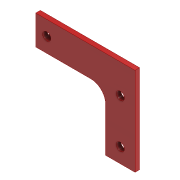
# Autodesk Inventor part: Odometry stop
Saved by Autodesk Inventor 2020 (Build 240168000, 168)
## iProperties
Created: 2020-03-07
Part Number: Odometry stop
Material: Generic
Document SubType Name: Modeling
Designer: ball
Density: 1 g/cm^3
Appearance: Default
Author: ball
Autodesk Inventor part; units mm, degrees
ref_plane "YZ Plane" through (0, 0, 0) normal (1, 0, 0) x (0, 1, 0)
ref_plane "XZ Plane" through (0, 0, 0) normal (0, 1, 0) x (-1, 0, 0)
ref_plane "XY Plane" through (0, 0, 0) normal (0, 0, 1) x (1, 0, 0)
ref_plane "Work Plane5" through (0, 0, 0) normal (0, 0, 1) x (1, 0, 0)
sketch "Sketch1" plane through (0, 0, 0) normal (0, 0, 1) x (1, 0, 0)
  arc A0 (-50, 35.3137) -> (-46, 35.3137) centre (-48, 35.3137) ccw construction
  arc A1 (-46, 40) -> (-50, 40) centre (-48, 40) ccw construction
  line L0 (-50, 35.3137) -> (-50, 40) construction
  line L1 (-46, 40) -> (-46, 35.3137) construction
  line L2 (-46.254, 38.8332) -> (-46.254, 35.3137)
  arc A2 (-49.746, 35.3137) -> (-46.254, 35.3137) centre (-48, 35.3137) ccw
  line L3 (-49.746, 35.3137) -> (-49.746, 38.8332)
  arc A3 (-49.746, 38.8332) -> (-46.254, 38.8332) centre (-48, 40) ccw
  point P0 (0, 0)
  dimension "d1" = 4.2
  constraints: 4 end point, 4 point on circle, 2 centre point, 1 coincident
  measures "d1" diameter of A3
extrude "Extrusion1" add sketch "Sketch1" against normal blind 2.5
ref_plane "Work Plane6" through (0, 0, 0) normal (0, 0, 1) x (1, 0, 0)
sketch "Sketch2" plane through (0, 0, 0) normal (0, 0, 1) x (1, 0, 0)
  line L0 (0, 48) -> (-192, 48) construction
  line L1 (-54, 45.5) -> (-54, 48) construction
  line L2 (-54, 48) -> (0, 48)
  line L3 (0, 48) -> (0, 0)
  line L4 (-54, 32) -> (-54, 48)
  arc A0 (-16, 24) -> (-24, 32) centre (-24, 24) ccw
  circle A1 centre (-8, 8) radius 2.2
  circle A2 centre (-8, 32) radius 2.2
  line L5 (-54, 32) -> (-24, 32)
  line L6 (-16, 24) -> (-16, 0)
  line L7 (0, 0) -> (-16, 0)
  dimension "d7" = 4.4
  dimension "d8" = 4.4
  dimension "d9" = 24
  constraints: 14 end point, 3 centre point, 2 coincident, 2 horizontal, 2 point on circle, 2 tangent, 1 parallel, 1 perpendicular, 1 vertical, 2 other
  measures "d7" diameter of A1
  measures "d8" diameter of A2
  measures "d9" distance of A2.centre point (-8, 8)
extrude "Extrusion2" add sketch "Sketch2" along normal blind 2.5
sketch "Sketch4" plane through (0, 0, -2.5) normal (0, 0, -1) x (-1, 0, 0)
  arc A0 (46.254, 38.8332) -> (49.746, 38.8332) centre (48, 40) ccw projected
  circle A1 centre (48, 40) radius 2.2
  point P0 (0, 0)
  dimension "d16" = 4.4
  constraints: 1 centre point, 1 coincident
  measures "d16" diameter of A1
extrude "Extrusion4" cut sketch "Sketch4" against normal through all
body "Solid1"
